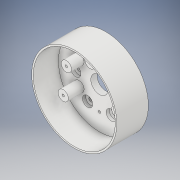
# Autodesk Inventor part: Base
Saved by Autodesk Inventor 2017 SP1 (Build 210196100, 196)
## iProperties
Created: 2017-09-22
Part Number: Base
Material: ABS Plastic
Document SubType Name: Modeling
Designer: Zach
Density: 1.06 g/cm^3
Appearance: CR White
Author: Zach
Autodesk Inventor part; units mm, degrees
ref_plane "YZ Plane" through (0, 0, 0) normal (1, 0, 0) x (0, 1, 0)
ref_plane "XZ Plane" through (0, 0, 0) normal (0, 1, 0) x (-1, 0, 0)
ref_plane "XY Plane" through (0, 0, 0) normal (0, 0, 1) x (1, 0, 0)
sketch "Sketch1" plane through (0, 0, 0) normal (0, 0, 1) x (1, 0, 0)
  circle A0 centre (0, 0) radius 54
  dimension "d0" = 108
  constraints: 1 centre point, 1 coincident
  measures "d0" diameter of A0
extrude "Extrusion1" add sketch "Sketch1" along normal blind 37
sketch "Sketch2" plane through (0, 0, 37) normal (0, 0, 1) x (1, 0, 0)
  circle A0 centre (0, 0) radius 54 projected
  circle A1 centre (0, 0) radius 52
  dimension "d3" = 2
  constraints: 1 centre point
  measures "d3" radial gap between concentric circles of A0 A1
extrude "Extrusion2" cut sketch "Sketch2" against normal blind 29 contours A1
sketch "Sketch3" plane through (0, 0, 8) normal (0, 0, 1) x (1, 0, 0)
  circle A0 centre (0, 0) radius 11
  dimension "d6" = 22
  constraints: 1 centre point, 1 coincident
  measures "d6" diameter of A0
extrude "Extrusion3" cut sketch "Sketch3" against normal through all
sketch "Sketch4" plane through (0, 0, 8) normal (0, 0, 1) x (1, 0, 0)
  circle A0 centre (30, 0) radius 6.5
  circle A1 centre (15, 25.9808) radius 6.5
  circle A2 centre (-15, 25.9808) radius 6.5
  circle A3 centre (-30, 0) radius 6.5
  circle A4 centre (-15, -25.9808) radius 6.5
  circle A5 centre (15, -25.9808) radius 6.5
  point P0 (0, 0)
  dimension "d9" = 13
  dimension "d10" = 30
  dimension "d13" = 360
  constraints: 6 centre point, 1 horizontal alignment, 13 other
  measures "d9" diameter of A0
  measures "d10" distance of point (0, 0) A0.centre
extrude "Extrusion4" cut sketch "Sketch4" against normal blind 4
sketch "Sketch5" plane through (0, 0, 8) normal (0, 0, 1) x (1, 0, 0)
  circle A0 centre (-15, -25.9808) radius 6.5 construction
  circle A1 centre (-15, 25.9808) radius 6.5 construction
  circle A2 centre (30, 0) radius 6.5 construction
  circle A3 centre (15, 25.9808) radius 6.5 construction
  circle A4 centre (-30, 0) radius 6.5 construction
  circle A5 centre (15, -25.9808) radius 6.5 construction
  circle A6 centre (0, 0) radius 11 construction
  circle A7 centre (0, 0) radius 52 construction
  circle A8 centre (30, 0) radius 2.5
  circle A9 centre (15, 25.9808) radius 2.5
  circle A10 centre (-15, 25.9808) radius 2.5
  circle A11 centre (-30, 0) radius 2.5
  circle A12 centre (-15, -25.9808) radius 2.5
  circle A13 centre (15, -25.9808) radius 2.5
  dimension "d17" = 5
  dimension "d20" = 360
  constraints: 14 centre point, 6 coincident, 19 other
  measures "d17" diameter of A8
extrude "Extrusion5" cut sketch "Sketch5" against normal through all
sketch "Sketch6" plane through (0, 0, 8) normal (0, 0, 1) x (1, 0, 0)
  circle A0 centre (0, 30) radius 1.5
  circle A1 centre (-25.9808, 15) radius 1.5
  circle A2 centre (-25.9808, -15) radius 1.5
  circle A3 centre (0, -30) radius 1.5
  circle A4 centre (25.9808, -15) radius 1.5
  circle A5 centre (25.9808, 15) radius 1.5
  point P0 (0, 0)
  dimension "d24" = 3
  dimension "d25" = 30
  dimension "d28" = 360
  constraints: 6 centre point, 1 vertical alignment, 13 other
  measures "d24" diameter of A0
  measures "d25" distance of point (0, 0) A0.centre
extrude "Extrusion6" cut sketch "Sketch6" against normal through all
sketch "Sketch7" plane through (0, 0, 8) normal (0, 0, 1) x (1, 0, 0)
  circle A0 centre (25.9808, -15) radius 1.5 projected
  circle A1 centre (25.9808, -15) radius 1.5 projected
  circle A2 centre (25.9808, -15) radius 6.5
  point P0 (0, 0)
  dimension "d32" = 13
  constraints: 1 centre point, 1 coincident
  measures "d32" diameter of A2
extrude "Extrusion7" add sketch "Sketch7" along normal blind 4
sketch "Sketch8" plane through (0, 0, 8) normal (0, 0, 1) x (1, 0, 0)
  circle A0 centre (25.9808, 15) radius 1.5 projected
  circle A1 centre (25.9808, 15) radius 6.5
  point P0 (0, 0)
  dimension "d35" = 13
  constraints: 1 centre point, 1 coincident
  measures "d35" diameter of A1
extrude "Extrusion8" add sketch "Sketch8" along normal blind 8
sketch "Sketch9" plane through (0, 0, 8) normal (0, 0, 1) x (1, 0, 0)
  circle A0 centre (0, 30) radius 1.5 projected
  circle A1 centre (0, 30) radius 6.5
  point P0 (0, 0)
  dimension "d38" = 13
  constraints: 1 centre point, 1 coincident
  measures "d38" diameter of A1
extrude "Extrusion9" add sketch "Sketch9" along normal blind 12
sketch "Sketch10" plane through (0, 0, 8) normal (0, 0, 1) x (1, 0, 0)
  circle A0 centre (-25.9808, 15) radius 1.5 projected
  circle A1 centre (-25.9808, 15) radius 6.5
  point P0 (0, 0)
  dimension "d41" = 13
  constraints: 1 centre point, 1 coincident
  measures "d41" diameter of A1
extrude "Extrusion10" add sketch "Sketch10" along normal blind 16
sketch "Sketch11" plane through (0, 0, 8) normal (0, 0, 1) x (1, 0, 0)
  circle A0 centre (-25.9808, -15) radius 1.5 projected
  circle A1 centre (-25.9808, -15) radius 6.5
  point P0 (0, 0)
  dimension "d44" = 13
  constraints: 1 centre point, 1 coincident
  measures "d44" diameter of A1
extrude "Extrusion11" add sketch "Sketch11" along normal blind 20
sketch "Sketch15" plane through (0, 0, 37) normal (0, 0, 1) x (1, 0, 0)
  circle A0 centre (0, 0) radius 52 projected
  circle A1 centre (0, 0) radius 54 projected
extrude "Extrusion15" add sketch "Sketch15" along normal blind 3
body "Solid1"
